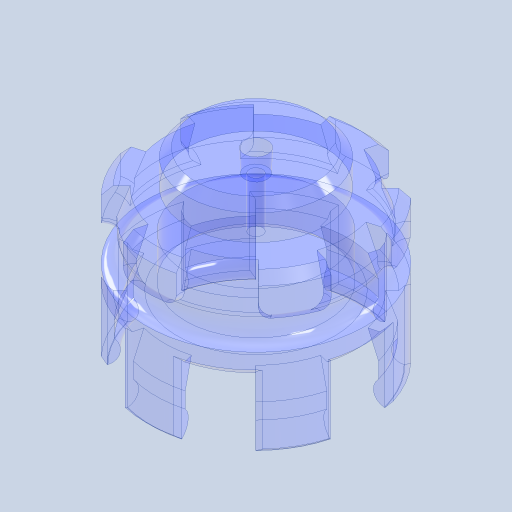
# Autodesk Inventor part: cpd_ultra-TLA100.3_0.7_p2_20230615
Saved by Autodesk Inventor 2024 (Build 280153000, 153)
## iProperties
Created: 2022-02-17
Part Number: cpd_ultra-TLA100.3_0.7_p2_20230615
Material: Generic
Document SubType Name: Modeling
Designer: to172
Density: 1 g/cm^3
Appearance: Clear - Blue
Author: to172
Autodesk Inventor part; units mm, degrees
ref_plane "YZ Plane" through (0, 0, 0) normal (1, 0, 0) x (0, 1, 0)
ref_plane "XZ Plane" through (0, 0, 0) normal (0, 1, 0) x (-1, 0, 0)
ref_plane "XY Plane" through (0, 0, 0) normal (0, 0, 1) x (1, 0, 0)
sketch "Sketch1" plane through (0, 0, 0) normal (0, 0, 1) x (1, 0, 0)
  line L0 (0, 0) -> (0, 2.282) construction
  line L1 (0, 0) -> (1.8038, 0) construction
  line L2 (0.3875, 0) -> (0.3875, 2.95)
  line L3 (0.3875, 2.95) -> (0.65, 2.95)
  line L4 (0.3875, 0) -> (4.1, 0)
  line L5 (4.1, 0) -> (4.1, -3)
  line L6 (4.1, -3) -> (6.4, -3)
  line L7 (4, 4.25) -> (4, 2.25)
  line L8 (4, 2.25) -> (6.4, 2.25)
  line L9 (6.4, 2.25) -> (6.4, -3)
  line L10 (0.65, 2.95) -> (0.6954, 4.25)
  line L11 (0.6954, 4.25) -> (4, 4.25)
  dimension "d0" = 0.3875
  dimension "d5" = 3
  dimension "d6" = 4.1
  dimension "d8" = 4
  dimension "d11" = 2
  dimension "d12" = 1.3
  dimension "d13" = 0.65
  dimension "d14" = 4.25
  dimension "d15" = 2
  dimension "d16" = 6.4
  constraints: 24 end point, 5 perpendicular, 3 vertical, 2 point on line, 1 horizontal
  measures "d0" distance between parallel lines of L2 L0
  measures "d5" distance between parallel lines of L1 L6
  measures "d6" distance between parallel lines of L5 L0
  measures "d8" distance between parallel lines of L7 L0
  measures "d11" angle of L0 L10
  measures "d12" distance between parallel lines of L11 L3
  measures "d13" distance from line of L3.end L0
  measures "d14" distance between parallel lines of L11 L1
  measures "d15" distance between parallel lines of L11 L8
  measures "d16" distance between parallel lines of L9 L0
revolve "Revolution1" add sketch "Sketch1" angle 360 about axis through (0, 0, 0) along (0, 1, 0)
sketch "Sketch2" plane through (0, 0, 0) normal (1, 0, 0) x (0, 1, 0)
  line L0 (0, 0) -> (-6.7378, 0) construction
  line L1 (0, 0) -> (0, -9.3136) construction
  line L2 (-3, 6.4) -> (-3, -6.4) construction
  line L3 (-3, 0) -> (-3, -10.17) construction
  line L4 (-3, -6.4) -> (-6.75, -6.4)
  line L5 (-6.75, -6.4) -> (-6.75, -5.85)
  line L6 (-6.75, -5.85) -> (-3, -5.85)
  line L7 (-3, -5.85) -> (-3, -6.4)
  line L8 (-8.16, 0) -> (1.36, 0) projected
  circle A0 centre (-6, -6.4) radius 0.8
  line L9 (-4.5, -5.85) -> (-3, -5.35)
  line L10 (-3, -5.35) -> (-3, -5.85)
  point P0 (-5.4191, -5.85)
  point P1 (-6.75, -6.1216)
  dimension "d18" = 0.55
  dimension "d44" = 1.6
  dimension "d45" = 3.75
  dimension "d46" = 0.75
  dimension "d47" = 0.5
  dimension "d48" = 1.5
  constraints: 18 end point, 3 point on line, 2 horizontal, 2 parallel, 2 vertical, 1 centre point, 1 collinear, 1 midpoint, 1 perpendicular
  measures "d18" distance between parallel lines of L4 L6
  measures "d44" diameter of A0
  measures "d45" distance between parallel lines of L3 L5
  measures "d46" distance from line of L5 A0.centre
  measures "d47" distance from line of L9.end L6
  measures "d48" distance of L6.end L9.start
revolve "Revolution2" add sketch "Sketch2" angle 30 mid plane about axis through (0, -10, 0) along (0, 1, 0) contours L4 A0 L6 L7 | L4 L5 A0 L6 | L6 L9 L10 | L6 A0
chamfer "Chamfer1" distance 0.25 angle 45 3 edges at (1.6564, -4.875, -6.1819) (-1.6564, -4.875, -6.1819) (0, -6.75, -6.4)
pattern_circular "Circular Pattern2" count 6 over 360 about axis through (0, -10, 0) along (0, 1, 0) of "Revolution2", "Chamfer1"
chamfer "Chamfer2" distance 0.5 angle 45 20 edges at (4.613, -3, -4.4362) (3.0911, -3, -5.604) (6.1484, -3, -1.7769) (6.3452, -3, -0.8354) (6.3452, -3, 0.8354) (6.1484, -3, 1.7769) (4.613, -3, 4.4362) (3.2, -3, 5.5426) (1.5354, -3, 6.2131) (-1.5354, -3, 6.2131) (-3.2, -3, 5.5426) (-4.613, -3, 4.4362) (-6.1484, -3, -1.7769) (-6.4, -3, 0) (-6.1484, -3, 1.7769) (-3.0911, -3, -5.604) (-4.613, -3, -4.4362) (-6.4, 2.25, 0) (-4, 4.25, 0) (-4.1, -3, 0)
sketch "Sketch3" plane through (0, 0, 0) normal (0, 0, 1) x (0, 1, 0)
  line L0 (0, 0) -> (0, -9.9283) construction
  line L1 (0, 4.1) -> (0, -4.1) construction
  line L2 (0, 0) -> (10.6094, 0) construction
  line L3 (2.25, 4) -> (2.25, -4) construction
  line L4 (2.25, 0) -> (2.25, -7.885) construction
  line L5 (1.75, -6.4) -> (-2.5, -6.4) projected
  circle A0 centre (-0.75, -6.4) radius 0.85
  line L6 (2.25, -6.4) -> (-0.75, -6.4)
  line L7 (-0.75, -6.4) -> (2.25, -6.4)
  line L8 (2.25, -6.4) -> (2.25, -5.75)
  line L9 (2.25, -5.75) -> (-0.75, -5.75)
  line L10 (-0.75, -5.75) -> (-0.75, -6.4)
  line L11 (-5.1219, 0) -> (13.2313, 0) projected
  line L12 (0.7, -5.75) -> (2.25, -5.2)
  line L13 (2.25, 5.9) -> (2.25, -5.9) projected
  line L14 (2.25, -5.2) -> (2.25, -5.75)
  point P0 (-1.6, -6.4)
  point P1 (0.1, -6.4)
  dimension "d34" = 1.7
  dimension "d35" = 3
  dimension "d36" = 0.65
  dimension "d49" = 0.55
  dimension "d50" = 1.55
  constraints: 20 end point, 5 point on line, 4 collinear, 2 horizontal, 2 parallel, 1 centre point, 1 midpoint, 1 perpendicular
  measures "d34" diameter of A0
  measures "d35" distance between parallel lines of L4 L10
  measures "d36" distance between parallel lines of L9 L6
  measures "d49" distance from line of L12.end L9
  measures "d50" distance from line of L14 L12.start
revolve "Revolution3" cut sketch "Sketch3" angle 360 about axis through (0, 0, 0) along (0, 1, 0) contours L5 L10 L9 A0 | L5 A0 L9 L10
revolve "Revolution4" cut sketch "Sketch3" angle 32 mid plane about axis through (0, -10, 0) along (0, 1, 0) picked at (-0.5674, -5.9667) contours L5 A0 L9 L8 L6 | L5 L10 L9 A0 | L12 L13 L9
fillet "Fillet1" radius 0.5 4 edges at (5.694, -0.2023, 0.8002) (5.694, -0.2023, -0.8002) (5.8075, 0.0207, 1.6653) (5.8075, 0.0207, -1.6653)
pattern_circular "Circular Pattern3" count 6 over 360 about axis through (0, -10, 0) along (0, 1, 0) of "Revolution4", "Fillet1"
body "Solid1"
